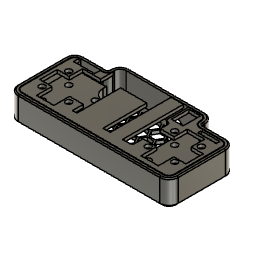
sprig_cover V7 v1 (Autodesk Fusion 360 design; units mm, degrees)
Autodesk Fusion 360 part; units mm, degrees
note: some values were not read from the file. Set by a fixed rule: which sketch regions a step uses.
(part 1 of 2)
sketch "Sketch2" plane through (0, 0, 0) normal (0, 0, 1) x (1, 0, 0)
  line L0 (65.104, -32.4032) -> (-65.104, -32.4032)
  line L1 (70.104, 16.1685) -> (70.104, -27.4032)
  line L2 (70.104, -32.4032) -> (77.8347, -35.9764) construction
  line L3 (12.9089, -32.4032) -> (70.104, -175.9712) construction
  arc A0 (-70.104, -27.4032) -> (-65.104, -32.4032) centre (-65.104, -27.4032) ccw
  line L4 (39.5875, 27.4935) -> (39.6132, 26.0776)
  line L5 (39.4501, 35.0437) -> (39.5, 32.512)
  line L6 (44.6124, 21.1685) -> (65.104, 21.1685)
  arc A1 (39.5875, 27.4935) -> (34.5883, 32.4025) centre (34.5883, 27.4025) ccw
  arc A2 (39.6132, 26.0776) -> (44.6124, 21.1685) centre (44.6124, 26.1685) ccw
  arc A3 (70.104, 16.1685) -> (65.104, 21.1685) centre (65.104, 16.1685) ccw
  arc A4 (65.104, -32.4032) -> (70.104, -27.4032) centre (65.104, -27.4032) ccw
  line L7 (0, 0) -> (0, 41.41)
  arc A5 (-44.6124, 21.1685) -> (-39.6132, 26.0776) centre (-44.6124, 26.1685) ccw
  line L8 (-44.6124, 21.1685) -> (-65.104, 21.1685)
  arc A6 (-65.104, 21.1685) -> (-70.104, 16.1685) centre (-65.104, 16.1685) ccw
  arc A7 (-34.5883, 32.4025) -> (-39.5875, 27.4935) centre (-34.5883, 27.4025) ccw
  line L9 (-39.5875, 27.4935) -> (-39.6132, 26.0776)
  line L10 (-34.5883, 32.4025) -> (34.5883, 32.4025)
  line L11 (-70.104, 16.1685) -> (-70.104, -27.4032)
  arc A8 (40.0874, 27.5026) -> (34.5883, 32.9025) centre (34.5883, 27.4025) ccw
  line L12 (-34.5883, 32.9025) -> (34.5883, 32.9025)
  arc A9 (-34.5883, 32.9025) -> (-40.0874, 27.5026) centre (-34.5883, 27.4025) ccw
  line L13 (-40.0874, 27.5026) -> (-40.1132, 26.0867)
  arc A10 (-44.6124, 21.6685) -> (-40.1132, 26.0867) centre (-44.6124, 26.1685) ccw
  line L14 (-44.6124, 21.6685) -> (-65.104, 21.6685)
  arc A11 (-65.104, 21.6685) -> (-70.604, 16.1685) centre (-65.104, 16.1685) ccw
  line L15 (-70.604, 16.1685) -> (-70.604, -27.4032)
  arc A12 (-70.604, -27.4032) -> (-65.104, -32.9032) centre (-65.104, -27.4032) ccw
  line L16 (65.104, -32.9032) -> (-65.104, -32.9032)
  arc A13 (65.104, -32.9032) -> (70.604, -27.4032) centre (65.104, -27.4032) ccw
  line L17 (70.604, 16.1685) -> (70.604, -27.4032)
  arc A14 (70.604, 16.1685) -> (65.104, 21.6685) centre (65.104, 16.1685) ccw
  line L18 (44.6124, 21.6685) -> (65.104, 21.6685)
  arc A15 (40.1132, 26.0867) -> (44.6124, 21.6685) centre (44.6124, 26.1685) ccw
  line L19 (40.0874, 27.5026) -> (40.1132, 26.0867)
  line L20 (-34.5883, 35.9025) -> (34.5883, 35.9025)
  arc A16 (43.0869, 27.5571) -> (34.5883, 35.9025) centre (34.5883, 27.4025) ccw
  line L21 (43.0869, 27.5571) -> (43.1127, 26.1412)
  arc A17 (43.1127, 26.1412) -> (44.6124, 24.6685) centre (44.6124, 26.1685) ccw
  line L22 (44.6124, 24.6685) -> (65.104, 24.6685)
  arc A18 (73.604, 16.1685) -> (65.104, 24.6685) centre (65.104, 16.1685) ccw
  line L23 (73.604, 16.1685) -> (73.604, -27.4032)
  arc A19 (65.104, -35.9032) -> (73.604, -27.4032) centre (65.104, -27.4032) ccw
  line L24 (65.104, -35.9032) -> (-65.104, -35.9032)
  arc A20 (-73.604, -27.4032) -> (-65.104, -35.9032) centre (-65.104, -27.4032) ccw
  line L25 (-73.604, 16.1685) -> (-73.604, -27.4032)
  arc A21 (-65.104, 24.6685) -> (-73.604, 16.1685) centre (-65.104, 16.1685) ccw
  line L26 (-44.6124, 24.6685) -> (-65.104, 24.6685)
  arc A22 (-44.6124, 24.6685) -> (-43.1127, 26.1412) centre (-44.6124, 26.1685) ccw
  line L27 (-43.0869, 27.5571) -> (-43.1127, 26.1412)
  arc A23 (-34.5883, 35.9025) -> (-43.0869, 27.5571) centre (-34.5883, 27.4025) ccw
  dimension "d1" = 140.208
  dimension "d2" = 65.024
  dimension "d58" = 5
  dimension "d59" = 5
  dimension "d60" = 5
  dimension "d61" = 5
  dimension "d62" = 5
  dimension "d63" = -0.5
  dimension "d64" = 3.5
  constraint horizontal L0
  constraint coincident L2 L7.start
  constraint coincident L3 L7.start
  constraint coincident L7.start origin
  constraint coincident L3.start L0
  constraint tangent L0 A0
  constraint perpendicular L1 L6
  constraint coincident L5.start L4
  constraint tangent L4 A1
  constraint tangent L4 A2
  constraint tangent L6 A2
  constraint coincident L3.end L1
  constraint tangent L6 A3
  constraint tangent L1 A3
  constraint coincident L2.start L0
  constraint coincident L2.start L1
  constraint tangent L0 A4
  constraint tangent L1 A4
  constraint symmetric A1.end L7 A7.start
  constraint symmetric L4.start L7 A7.end
  constraint symmetric A1 L7 A7
  constraint symmetric L4.end L7 A5.end
  constraint symmetric L6.start L7 A5.start
  constraint symmetric A2 L7 A5
  constraint symmetric L6.end L7 L8.end
  constraint symmetric L1.start L7 A6.end
  constraint symmetric A3 L7 A6
  constraint tangent A1 L10
  constraint tangent A0 L11
  measures "d1" distance of L2.end L3.end
  measures "d2" distance of L3.start L2.end
  measures "d58" radius of A0
  measures "d59" radius of A1
  measures "d60" radius of A2
  measures "d61" radius of A3
  measures "d62" radius of A4
sketch "Sketch3" plane through (0, 0, 0) normal (0, 0, 1) x (1, 0, 0)
  line L0 (-70.104, 15.8) -> (-70.104, -27.3)
  arc A0 (-70.104, -27.3) -> (-64.904, -32.5) centre (-64.904, -27.3) ccw
  line L1 (-64.904, -32.5) -> (-30, -32.5)
  arc A1 (-64.904, 21) -> (-70.104, 15.8) centre (-64.904, 15.8) ccw
  line L2 (-64.904, 21) -> (-42, 21)
  line L3 (-30, 9) -> (-30, -32.5)
  circle A2 centre (-30.5373, 18.3875) radius 8
  line L4 (-30.5373, 22.2562) -> (-30.5373, 14.5188)
  line L5 (-42, 21) -> (-42, 19)
  arc A3 (-42, 19) -> (-32, 9) centre (-32, 19) ccw
  line L6 (-32, 9) -> (-30, 9)
  line L7 (0, 0) -> (0, 41.41)
  line L8 (64.904, -32.5) -> (30, -32.5)
  line L9 (30, 9) -> (30, -32.5)
  arc A4 (32, 9) -> (42, 19) centre (32, 19) ccw
  line L10 (64.904, 21) -> (42, 21)
  line L11 (42, 21) -> (42, 19)
  line L12 (70.104, 15.8) -> (70.104, -27.3)
  arc A5 (70.104, 15.8) -> (64.904, 21) centre (64.904, 15.8) ccw
  arc A6 (64.904, -32.5) -> (70.104, -27.3) centre (64.904, -27.3) ccw
  line L13 (30, 9) -> (32, 9)
  line L14 (-64.904, -27.5) -> (-35, -27.5)
  line L15 (-35, 4.3031) -> (-35, -27.5)
  arc A7 (-46.6969, 16) -> (-35, 4.3031) centre (-32, 19) ccw
  line L16 (-64.904, 16) -> (-46.6969, 16)
  arc A8 (-64.904, 16) -> (-65.104, 15.8) centre (-64.904, 15.8) ccw
  line L17 (-65.104, 15.8) -> (-65.104, -27.3)
  arc A9 (-65.104, -27.3) -> (-64.904, -27.5) centre (-64.904, -27.3) ccw
  line L18 (64.904, -27.5) -> (35, -27.5)
  line L19 (35, 4.3031) -> (35, -27.5)
  arc A10 (35, 4.3031) -> (46.6969, 16) centre (32, 19) ccw
  line L20 (64.904, 16) -> (46.6969, 16)
  arc A11 (65.104, 15.8) -> (64.904, 16) centre (64.904, 15.8) ccw
  line L21 (65.104, 15.8) -> (65.104, -27.3)
  arc A12 (64.904, -27.5) -> (65.104, -27.3) centre (64.904, -27.3) ccw
  dimension "d3" = 70.104
  dimension "d4" = 32.5
  dimension "d5" = 5.2
  dimension "d6" = 21
  dimension "d7" = 5.2
  dimension "d8" = 16
  dimension "d9" = 42
  dimension "d10" = 9
  dimension "d11" = 10
  dimension "d12" = 30
  dimension "d97" = 5
  dimension "d98" = -5
  constraint vertical L0
  constraint tangent L0 A0
  constraint horizontal L1
  constraint tangent A0 L1
  constraint tangent L0 A1
  constraint horizontal L2
  constraint tangent A1 L2
  constraint perpendicular L2 L3
  constraint coincident L1.end L3.end
  constraint vertical L4
  constraint midpoint A2.centre L4
  constraint perpendicular L2 L5
  constraint tangent L5 A3
  constraint perpendicular L5 L6
  constraint tangent A3 L6
  constraint symmetric L0.start L7 L12.start
  constraint symmetric L0.end L7 L12.end
  constraint symmetric A0.end L7 L8.start
  constraint symmetric A0 L7 A6
  constraint symmetric L1.end L7 L8.end
  constraint symmetric A1.start L7 L10.start
  constraint symmetric A1 L7 A5
  constraint symmetric L2.end L7 L10.end
  constraint symmetric L5.end L7 A4.end
  constraint symmetric A3.end L7 A4.start
  constraint symmetric A3 L7 A4
  constraint symmetric L3.start L7 L9.start
  measures "d3" distance of L7.start L0
  measures "d4" distance of L7.start L1
  measures "d5" radius of A0
  measures "d6" distance of L7.start L2
  measures "d7" radius of A1
  measures "d8" diameter of A2
  measures "d9" distance of L7.start L5
  measures "d10" distance of L7.start L6
  measures "d11" radius of A3
  measures "d12" distance of L7.start L3
extrude "Extrude1" add sketch "Sketch3" against normal blind 4 contours L0 A0 L1 A1 L2 L3 L5 A3 L6 | L14 L15 A7 L16 A8 L17 A9 makes body 1
fillet "Fillet3" radius 1 3 edges at (-30, -32.5, -2) (-30, 9, -2) (-42, 21, -2) on bodies 1
pattern_linear "R-Pattern1" count 2 spacing 4 along (0, 0, -1) of bodies 1 makes body 2
sketch "Sketch4" plane through (0, 0, 0) normal (0, 0, 1) x (-1, 0, 0)
  arc A0 (64.904, -21) -> (70.104, -15.8) centre (64.904, -15.8) ccw
  line L0 (70.104, -15.8) -> (70.104, 27.3)
  arc A1 (70.104, 27.3) -> (64.904, 32.5) centre (64.904, 27.3) ccw
  line L1 (64.904, 32.5) -> (31, 32.5)
  line L2 (30, 31.5) -> (30, -8)
  line L3 (31, -9) -> (32, -9)
  arc A2 (42, -19) -> (32, -9) centre (32, -19) ccw
  line L4 (42, -19) -> (42, -20)
  line L5 (43, -21) -> (64.904, -21)
  line L6 (65.35, -2.7) -> (48.35, -2.7)
  line L7 (65.35, 14.3) -> (65.35, -2.7)
  arc A3 (42, -20) -> (43, -21) centre (43, -20) ccw
  arc A4 (31, 32.5) -> (30, 31.5) centre (31, 31.5) ccw
  arc A5 (30, -8) -> (31, -9) centre (31, -8) ccw
  point P0 (48.35, 5.8)
  dimension "d21" = 5.8
  dimension "d23" = 48.35
  dimension "d24" = 17
  constraint horizontal L6
  constraint vertical L7
  measures "d21" vertical distance of origin P0
  measures "d23" horizontal distance of origin P0
  measures "d24" distance of L6.start L7.start
sketch "Sketch5" plane through (0, 0, 0) normal (0, 0, 1) x (-1, 0, 0)
  arc A0 (42, -20) -> (43, -21) centre (43, -20) ccw
  line L0 (43, -21) -> (64.904, -21)
  arc A1 (64.904, -21) -> (70.104, -15.8) centre (64.904, -15.8) ccw
  line L1 (70.104, -15.8) -> (70.104, 27.3)
  arc A2 (70.104, 27.3) -> (64.904, 32.5) centre (64.904, 27.3) ccw
  line L2 (64.904, 32.5) -> (31, 32.5)
  arc A3 (31, 32.5) -> (30, 31.5) centre (31, 31.5) ccw
  line L3 (30, 31.5) -> (30, -8)
  arc A4 (30, -8) -> (31, -9) centre (31, -8) ccw
  line L4 (31, -9) -> (32, -9)
  arc A5 (42, -19) -> (32, -9) centre (32, -19) ccw
  line L5 (42, -19) -> (42, -20)
  line L6 (62.35, -2.7) -> (62.35, -15.2)
  line L7 (62.35, -15.2) -> (51.35, -15.2)
  line L8 (51.35, -15.2) -> (51.35, -2.7)
  point P0 (56.85, -2.7)
  point P1 (56.85, -15.2)
  dimension "d37" = 12.5
  dimension "d38" = 11
  constraint perpendicular L6 L7
  constraint midpoint L7 P1
  constraint vertical P0 P1
  measures "d37" distance of L7.end L8.end
  measures "d38" distance of L6.end L7.end
sketch "Sketch6" plane through (0, 0, 0) normal (0, 0, 1) x (-1, 0, 0)
  arc A0 (42, -20) -> (43, -21) centre (43, -20) ccw
  line L0 (43, -21) -> (64.904, -21)
  arc A1 (64.904, -21) -> (70.104, -15.8) centre (64.904, -15.8) ccw
  line L1 (70.104, -15.8) -> (70.104, 27.3)
  arc A2 (70.104, 27.3) -> (64.904, 32.5) centre (64.904, 27.3) ccw
  line L2 (64.904, 32.5) -> (31, 32.5)
  arc A3 (31, 32.5) -> (30, 31.5) centre (31, 31.5) ccw
  line L3 (30, 31.5) -> (30, -8)
  arc A4 (30, -8) -> (31, -9) centre (31, -8) ccw
  line L4 (31, -9) -> (32, -9)
  arc A5 (42, -19) -> (32, -9) centre (32, -19) ccw
  line L5 (42, -19) -> (42, -20)
  circle A6 centre (60.5272, -6.0993) radius 1.1
  circle A7 centre (36.0826, -6.0993) radius 1.1
  line L6 (60.5272, -6.0993) -> (36.0826, -6.0993) construction
  line L7 (36.0826, -6.0993) -> (36.0826, 18.3161) construction
  line L8 (36.0826, 18.3161) -> (60.5272, 18.3161) construction
  line L9 (60.5272, 18.3161) -> (60.5272, -6.0993) construction
  circle A8 centre (60.5272, 18.3161) radius 1.1
  circle A9 centre (36.0826, 18.3161) radius 1.1
  dimension "d45" = 2.2
  dimension "d46" = 2.2
  dimension "d47" = 2.2
  dimension "d48" = 2.2
  constraint horizontal L6
  constraint vertical L7
  constraint horizontal L8
  constraint vertical L9
  constraint coincident A6.centre L6.start
  constraint coincident A7.centre L6.end
  constraint coincident L8.end L9.start
  constraint coincident L7.end L8.start
  measures "d45" diameter of A6
  measures "d46" diameter of A7
  measures "d47" diameter of A8
  measures "d48" diameter of A9
sketch "Sketch10" plane through (0, 0, 0) normal (0, 0, 1) x (-1, 0, 0)
  arc A0 (42, -20) -> (43, -21) centre (43, -20) ccw
  line L0 (43, -21) -> (64.904, -21)
  arc A1 (64.904, -21) -> (70.104, -15.8) centre (64.904, -15.8) ccw
  line L1 (70.104, -15.8) -> (70.104, 27.3)
  arc A2 (70.104, 27.3) -> (64.904, 32.5) centre (64.904, 27.3) ccw
  line L2 (64.904, 32.5) -> (31, 32.5)
  arc A3 (31, 32.5) -> (30, 31.5) centre (31, 31.5) ccw
  line L3 (30, 31.5) -> (30, -8)
  arc A4 (30, -8) -> (31, -9) centre (31, -8) ccw
  line L4 (31, -9) -> (32, -9)
  arc A5 (42, -19) -> (32, -9) centre (32, -19) ccw
  line L5 (42, -19) -> (42, -20)
sketch "Sketch11" plane through (0, 0, -4) normal (0, 0, 1) x (-1, 0, 0)
  arc A0 (42, -20) -> (43, -21) centre (43, -20) ccw
  line L0 (43, -21) -> (64.904, -21)
  arc A1 (64.904, -21) -> (70.104, -15.8) centre (64.904, -15.8) ccw
  line L1 (70.104, -15.8) -> (70.104, 27.3)
  arc A2 (70.104, 27.3) -> (64.904, 32.5) centre (64.904, 27.3) ccw
  line L2 (64.904, 32.5) -> (31, 32.5)
  arc A3 (31, 32.5) -> (30, 31.5) centre (31, 31.5) ccw
  line L3 (30, 31.5) -> (30, -8)
  arc A4 (30, -8) -> (31, -9) centre (31, -8) ccw
  line L4 (31, -9) -> (32, -9)
  arc A5 (42, -19) -> (32, -9) centre (32, -19) ccw
  line L5 (42, -19) -> (42, -20)
extrude "Extrude7" add sketch "Sketch2" along normal blind 7 separate body contours L20 A16 L21 A17 L22 A18 L23 A19 L24 A20 L25 A21 L26 A22 L27 A23 makes body 3
extrude "Extrude8" add 1 faces at (-21.7013, -33.9032, 0) along direction (0, 0, -1) blind 18 separate body on bodies 3 makes body 4
extrude "Extrude9" add sketch "Sketch3" against normal blind 7.75 separate body contours A2 makes body 5
sketch "Sketch12" plane through (0, 0, -18) normal (0, 0, -1) x (1, 0, 0)
  arc A0 (-40.0874, -27.5026) -> (-34.5883, -32.9025) centre (-34.5883, -27.4025) ccw
  line L0 (-40.0874, -27.5026) -> (-40.1132, -26.0867)
  arc A1 (-40.1132, -26.0867) -> (-44.6124, -21.6685) centre (-44.6124, -26.1685) ccw
  line L1 (-44.6124, -21.6685) -> (-65.104, -21.6685)
  arc A2 (-70.604, -16.1685) -> (-65.104, -21.6685) centre (-65.104, -16.1685) ccw
  line L2 (-70.604, -16.1685) -> (-70.604, 27.4032)
  arc A3 (-65.104, 32.9032) -> (-70.604, 27.4032) centre (-65.104, 27.4032) ccw
  line L3 (-65.104, 32.9032) -> (65.104, 32.9032)
  arc A4 (70.604, 27.4032) -> (65.104, 32.9032) centre (65.104, 27.4032) ccw
  line L4 (70.604, 27.4032) -> (70.604, -16.1685)
  arc A5 (65.104, -21.6685) -> (70.604, -16.1685) centre (65.104, -16.1685) ccw
  line L5 (65.104, -21.6685) -> (44.6124, -21.6685)
  arc A6 (44.6124, -21.6685) -> (40.1132, -26.0867) centre (44.6124, -26.1685) ccw
  line L6 (40.1132, -26.0867) -> (40.0874, -27.5026)
  arc A7 (34.5883, -32.9025) -> (40.0874, -27.5026) centre (34.5883, -27.4025) ccw
  line L7 (34.5883, -32.9025) -> (-34.5883, -32.9025)
  arc A8 (34.5883, -35.9025) -> (43.0869, -27.5571) centre (34.5883, -27.4025) ccw
  line L8 (43.0869, -27.5571) -> (43.1127, -26.1412)
  arc A9 (44.6124, -24.6685) -> (43.1127, -26.1412) centre (44.6124, -26.1685) ccw
  line L9 (44.6124, -24.6685) -> (65.104, -24.6685)
  arc A10 (65.104, -24.6685) -> (73.604, -16.1685) centre (65.104, -16.1685) ccw
  line L10 (73.604, -16.1685) -> (73.604, 27.4032)
  arc A11 (73.604, 27.4032) -> (65.104, 35.9032) centre (65.104, 27.4032) ccw
  line L11 (65.104, 35.9032) -> (-65.104, 35.9032)
  arc A12 (-65.104, 35.9032) -> (-73.604, 27.4032) centre (-65.104, 27.4032) ccw
  line L12 (-73.604, 27.4032) -> (-73.604, -16.1685)
  arc A13 (-73.604, -16.1685) -> (-65.104, -24.6685) centre (-65.104, -16.1685) ccw
  line L13 (-65.104, -24.6685) -> (-44.6124, -24.6685)
  arc A14 (-43.1127, -26.1412) -> (-44.6124, -24.6685) centre (-44.6124, -26.1685) ccw
  line L14 (-43.1127, -26.1412) -> (-43.0869, -27.5571)
  arc A15 (-43.0869, -27.5571) -> (-34.5883, -35.9025) centre (-34.5883, -27.4025) ccw
  line L15 (-34.5883, -35.9025) -> (34.5883, -35.9025)
  line L16 (65.104, 35.9032) -> (-65.104, 35.9032)
  arc A16 (-65.104, 35.9032) -> (-73.604, 27.4032) centre (-65.104, 27.4032) ccw
  line L17 (-73.604, -16.1685) -> (-73.604, 27.4032)
  arc A17 (-73.604, -16.1685) -> (-65.104, -24.6685) centre (-65.104, -16.1685) ccw
  line L18 (-44.6124, -24.6685) -> (-65.104, -24.6685)
  line L19 (-34.5883, -35.9025) -> (34.5883, -35.9025)
  arc A18 (-43.0869, -27.5571) -> (-34.5883, -35.9025) centre (-34.5883, -27.4025) ccw
  arc A19 (-43.1127, -26.1412) -> (-44.6124, -24.6685) centre (-44.6124, -26.1685) ccw
  line L20 (-43.0869, -27.5571) -> (-43.1127, -26.1412)
  arc A20 (34.5883, -35.9025) -> (43.0869, -27.5571) centre (34.5883, -27.4025) ccw
  line L21 (44.6124, -24.6685) -> (65.104, -24.6685)
  line L22 (43.0869, -27.5571) -> (43.1127, -26.1412)
  arc A21 (44.6124, -24.6685) -> (43.1127, -26.1412) centre (44.6124, -26.1685) ccw
  arc A22 (65.104, -24.6685) -> (73.604, -16.1685) centre (65.104, -16.1685) ccw
  line L23 (73.604, -16.1685) -> (73.604, 27.4032)
  arc A23 (73.604, 27.4032) -> (65.104, 35.9032) centre (65.104, 27.4032) ccw
extrude "Extrude10" add sketch "Sketch12" along normal blind 3 separate body contours A0 L0 A1 L1 A2 L2 A3 L3 A4 L4 A5 L5 A6 L6 A7 L7 | A8 L8 A9 L9 A10 L10 A11 L11 A12 L12 A13 L13 A14 L14 A15 L15 L16 A16 L17 A17 L18 L19 A18 A19 L20 A20 L21 L22 A21 A22 L23 A23 makes body 6
sketch "Sketch13" plane through (0, 0, -8) normal (0, 0, -1) x (1, 0, 0)
  arc A0 (-43, -21) -> (-42, -20) centre (-43, -20) ccw
  line L0 (-42, -20) -> (-42, -19)
  arc A1 (-32, -9) -> (-42, -19) centre (-32, -19) ccw
  line L1 (-32, -9) -> (-31, -9)
  arc A2 (-31, -9) -> (-30, -8) centre (-31, -8) ccw
  line L2 (-30, -8) -> (-30, 31.5)
  arc A3 (-30, 31.5) -> (-31, 32.5) centre (-31, 31.5) ccw
  line L3 (-31, 32.5) -> (-64.904, 32.5)
  arc A4 (-64.904, 32.5) -> (-70.104, 27.3) centre (-64.904, 27.3) ccw
  line L4 (-70.104, 27.3) -> (-70.104, -15.8)
  arc A5 (-70.104, -15.8) -> (-64.904, -21) centre (-64.904, -15.8) ccw
  line L5 (-64.904, -21) -> (-43, -21)
  line L6 (0, -40) -> (0, 40)
  line L7 (42, -20) -> (42, -19)
  arc A6 (30, -8) -> (31, -9) centre (31, -8) ccw
  line L8 (70.104, 27.3) -> (70.104, -15.8)
  arc A7 (42, -20) -> (43, -21) centre (43, -20) ccw
  line L9 (32, -9) -> (31, -9)
  line L10 (30, -8) -> (30, 31.5)
  line L11 (31, 32.5) -> (64.904, 32.5)
  arc A8 (70.104, 27.3) -> (64.904, 32.5) centre (64.904, 27.3) ccw
  arc A9 (31, 32.5) -> (30, 31.5) centre (31, 31.5) ccw
  arc A10 (64.904, -21) -> (70.104, -15.8) centre (64.904, -15.8) ccw
  line L12 (64.904, -21) -> (43, -21)
  arc A11 (42, -19) -> (32, -9) centre (32, -19) ccw
  line L13 (30, -8) -> (30, -32.9025)
  line L14 (-34.5883, -32.4025) -> (34.5883, -32.4025)
  arc A12 (34.5883, -32.4025) -> (39.5875, -27.4935) centre (34.5883, -27.4025) ccw
  arc A13 (44.6124, -21.1685) -> (39.6132, -26.0776) centre (44.6124, -26.1685) ccw
  line L15 (39.5875, -27.4935) -> (39.6132, -26.0776)
  line L16 (42, -19.5) -> (42, -21.9053)
  line L17 (45.6567, -21) -> (44.6124, -21.1685)
  arc A14 (-40.0874, -27.5026) -> (-34.5883, -32.9025) centre (-34.5883, -27.4025) ccw
  line L18 (-34.5883, -32.9025) -> (34.5883, -32.9025)
  arc A15 (34.5883, -32.9025) -> (40.0874, -27.5026) centre (34.5883, -27.4025) ccw
  line L19 (40.0874, -27.5026) -> (40.1132, -26.0867)
  arc A16 (44.6124, -21.6685) -> (40.1132, -26.0867) centre (44.6124, -26.1685) ccw
  line L20 (44.6124, -21.6685) -> (65.104, -21.6685)
  arc A17 (65.104, -21.6685) -> (70.604, -16.1685) centre (65.104, -16.1685) ccw
  line L21 (70.604, -16.1685) -> (70.604, 27.4032)
  arc A18 (70.604, 27.4032) -> (65.104, 32.9032) centre (65.104, 27.4032) ccw
  line L22 (65.104, 32.9032) -> (-65.104, 32.9032)
  arc A19 (-65.104, 32.9032) -> (-70.604, 27.4032) centre (-65.104, 27.4032) ccw
  line L23 (-70.604, 27.4032) -> (-70.604, -16.1685)
  arc A20 (-70.604, -16.1685) -> (-65.104, -21.6685) centre (-65.104, -16.1685) ccw
  line L24 (-65.104, -21.6685) -> (-44.6124, -21.6685)
  arc A21 (-40.1132, -26.0867) -> (-44.6124, -21.6685) centre (-44.6124, -26.1685) ccw
  line L25 (-40.1132, -26.0867) -> (-40.0874, -27.5026)
  arc A22 (34.5883, -35.9025) -> (43.0869, -27.5571) centre (34.5883, -27.4025) ccw
  line L26 (34.5883, -35.9025) -> (-34.5883, -35.9025)
  arc A23 (-43.0869, -27.5571) -> (-34.5883, -35.9025) centre (-34.5883, -27.4025) ccw
  line L27 (-43.0869, -27.5571) -> (-43.1127, -26.1412)
  arc A24 (-43.1127, -26.1412) -> (-44.6124, -24.6685) centre (-44.6124, -26.1685) ccw
  line L28 (-44.6124, -24.6685) -> (-65.104, -24.6685)
  arc A25 (-73.604, -16.1685) -> (-65.104, -24.6685) centre (-65.104, -16.1685) ccw
  line L29 (-73.604, -16.1685) -> (-73.604, 27.4032)
  arc A26 (-65.104, 35.9032) -> (-73.604, 27.4032) centre (-65.104, 27.4032) ccw
  line L30 (-65.104, 35.9032) -> (65.104, 35.9032)
  arc A27 (73.604, 27.4032) -> (65.104, 35.9032) centre (65.104, 27.4032) ccw
  line L31 (73.604, 27.4032) -> (73.604, -16.1685)
  arc A28 (65.104, -24.6685) -> (73.604, -16.1685) centre (65.104, -16.1685) ccw
  line L32 (65.104, -24.6685) -> (44.6124, -24.6685)
  arc A29 (44.6124, -24.6685) -> (43.1127, -26.1412) centre (44.6124, -26.1685) ccw
  line L33 (43.1127, -26.1412) -> (43.0869, -27.5571)
  line L34 (-42, -19) -> (-42, -22.5045)
  line L35 (-30, 31.5) -> (-30, 32.9032)
  line L36 (30, 31.5) -> (30, 32.9032)
  constraint vertical L6
  constraint symmetric A0.start L6 A7.end
  constraint symmetric A0.end L6 L7.start
  constraint symmetric A0 L6 A7
  constraint symmetric L0.end L6 L7.end
  constraint symmetric A1.start L6 L9.start
  constraint symmetric A1 L6 A11
  constraint symmetric L1.end L6 A6.end
  constraint symmetric A2.end L6 A6.start
  constraint symmetric A2 L6 A6
  constraint symmetric L2.end L6 L10.end
  constraint symmetric A3.end L6 L11.start
  constraint symmetric A3 L6 A9
  constraint symmetric L3.end L6 L11.end
  constraint symmetric A4.end L6 L8.start
  constraint symmetric A4 L6 A8
  constraint symmetric L4.end L6 L8.end
  constraint symmetric A5.end L6 A10.start
  constraint symmetric A5 L6 A10
  constraint tangent A6 L13
  constraint midpoint L7 L16.start
  constraint coincident A13 L16.end
  constraint parallel L7 L16
  constraint coincident L12 L17.start
  constraint coincident A13.start L17.end
  constraint coincident L0.end A1.end
  constraint coincident A21 L34.end
  constraint tangent A1 L34
  constraint coincident L2.end A3.start
  constraint coincident L22 L35.end
  constraint tangent A3 L35
  constraint coincident L22 L36.end
  constraint tangent A9 L36
  constraint coincident L13.end L18
extrude "Extrude11" add sketch "Sketch13" along normal up to surface (10 mm away) separate body contours A0 L0 A1 L1 A2 L2 A3 L3 A4 L4 A5 L5 L34 | A0 A3 L3 A4 L4 A5 L5 L22 A19 L23 A20 L24 A21 L34 L35 | L8 L11 A8 A9 A10 L12 L13 L14 A12 A13 L15 L17 L18 A15 L19 A16 L20 A17 L21 A18 L22 L36 | L7 A6 L9 A11 L13 L14 A12 A13 L15 L16 | L7 A6 L8 A7 L9 L10 L11 A8 A9 A10 L12 A11 L16 | A7 L12 A13 L16 L17 makes body 7 at (-43.7527, -18.6342, -8) makes body 8 at (48.4055, -12.8793, -18)
sketch "Sketch15" plane through (0, 0, -8) normal (0, 0, 1) x (-1, 0, 0)
  arc A0 (-54.9753, -18.5428) -> (-41.9871, -20.3021) centre (-48.0353, -16.1308) ccw
  line L0 (-41.9871, -20.3021) -> (-41.9873, -19.0036)
  arc A1 (-32.0015, -9.0019) -> (-41.9873, -19.0036) centre (-31.9919, -18.9973) ccw
  line L1 (-32.0015, -9.0019) -> (-30.9998, -9.0018)
  arc A2 (-30.9998, -9.0018) -> (-29.9996, -8.0003) centre (-31.0003, -8.001) ccw
  line L2 (-29.9996, -8.0003) -> (-30.0003, 31.5)
  arc A3 (-30.0003, 31.5) -> (-31, 32.4989) centre (-30.9998, 31.4994) ccw
  line L3 (-31, 32.4989) -> (-64.904, 32.4966)
  arc A4 (-64.904, 32.4966) -> (-70.0751, 27.2999) centre (-64.8897, 27.3112) ccw
  line L4 (-70.0751, 27.2999) -> (-70.4263, -15.7823)
  arc A5 (-70.4263, -15.7823) -> (-55.331, -20.7119) centre (-62.9093, -18.3409) ccw
  line L5 (-55.331, -20.7119) -> (-54.9753, -18.5428)
  circle A6 centre (60.5404, -6.0319) radius 2.75
  circle A7 centre (36.0404, -6.0319) radius 2.75
  circle A8 centre (60.5404, 18.4681) radius 2.75
  circle A9 centre (36.0404, 18.4681) radius 2.75
  line L6 (0, 0) -> (0, -24.1722)
  circle A10 centre (-60.5404, 17.4681) radius 2.75
  circle A11 centre (-36.0404, 17.4681) radius 2.75
  circle A12 centre (-36.0404, -7.0319) radius 2.75
  circle A13 centre (-60.5404, -7.0319) radius 2.75
  line L7 (-30, -32.9025) -> (-30, 32.9032)
  line L8 (-30, -32.9025) -> (-30.1, -32.4)
  arc A14 (-39.5875, -27.4935) -> (-34.5883, -32.4025) centre (-34.5883, -27.4025) ccw
  line L9 (34.5883, -32.4025) -> (-34.5883, -32.4025)
  arc A15 (-39.6132, -26.0776) -> (-44.6124, -21.1685) centre (-44.6124, -26.1685) ccw
  line L10 (-39.5875, -27.4935) -> (-39.6132, -26.0776)
  line L11 (-45.6567, -21) -> (-43, -21.4357)
  line L12 (-30, 32.9032) -> (-65.104, 32.9032)
  arc A16 (-65.104, 32.9032) -> (-70.604, 27.4032) centre (-65.104, 27.4032) ccw
  line L13 (-70.604, 27.4032) -> (-70.604, -16.1685)
  arc A17 (-70.604, -16.1685) -> (-65.104, -21.6685) centre (-65.104, -16.1685) ccw
  line L14 (-65.104, -21.6685) -> (-44.6124, -21.6685)
  arc A18 (-40.1132, -26.0867) -> (-44.6124, -21.6685) centre (-44.6124, -26.1685) ccw
  line L15 (-40.1132, -26.0867) -> (-40.0874, -27.5026)
  arc A19 (-40.0874, -27.5026) -> (-34.5883, -32.9025) centre (-34.5883, -27.4025) ccw
  line L16 (-34.5883, -32.9025) -> (-30, -32.9025)
  dimension "d76" = 5.5
  dimension "d79" = -24.5
  dimension "d80" = 24.5
  constraint coincident L6.start origin
  constraint vertical L6
  constraint coincident L7.start L8.start
  constraint coincident A15 L11.end
  constraint perpendicular L5 L11
  measures "d76" diameter of A6
extrude "Extrude12" cut sketch "Sketch15" against normal blind 5 contours A1 A12 | A1 A12 | A6 | A7 | A8 | A9 | A10 | A11 | A13 bodies 7 8
sketch "Sketch16" plane through (0, 0, -21) normal (0, 0, -1) x (1, 0, 0)
  line L0 (44.6124, -24.6685) -> (65.104, -24.6685)
  arc A0 (65.104, -24.6685) -> (73.604, -16.1685) centre (65.104, -16.1685) ccw
  line L1 (73.604, -16.1685) -> (73.604, 27.4032)
  arc A1 (73.604, 27.4032) -> (65.104, 35.9032) centre (65.104, 27.4032) ccw
  line L2 (65.104, 35.9032) -> (-65.104, 35.9032)
  arc A2 (-65.104, 35.9032) -> (-73.604, 27.4032) centre (-65.104, 27.4032) ccw
  line L3 (-73.604, 27.4032) -> (-73.604, -16.1685)
  arc A3 (-73.604, -16.1685) -> (-65.104, -24.6685) centre (-65.104, -16.1685) ccw
  line L4 (-65.104, -24.6685) -> (-44.6124, -24.6685)
  arc A4 (-43.1127, -26.1412) -> (-44.6124, -24.6685) centre (-44.6124, -26.1685) ccw
  line L5 (-43.1127, -26.1412) -> (-43.0869, -27.5571)
  arc A5 (-43.0869, -27.5571) -> (-34.5883, -35.9025) centre (-34.5883, -27.4025) ccw
  line L6 (-34.5883, -35.9025) -> (34.5883, -35.9025)
  arc A6 (34.5883, -35.9025) -> (43.0869, -27.5571) centre (34.5883, -27.4025) ccw
  line L7 (43.0869, -27.5571) -> (43.1127, -26.1412)
  arc A7 (44.6124, -24.6685) -> (43.1127, -26.1412) centre (44.6124, -26.1685) ccw
  line L8 (-30, -8) -> (-30, 31.5)
  arc A8 (-32, -9) -> (-42, -19) centre (-32, -19) ccw
  line L9 (-43, -21) -> (-64.904, -21)
  arc A9 (-70.104, -15.8) -> (-64.904, -21) centre (-64.904, -15.8) ccw
  arc A10 (42, -19) -> (32, -9) centre (32, -19) ccw
  line L10 (30, -8) -> (30, 31.5)
  line L11 (64.904, -21) -> (43, -21)
  line L12 (70.104, 27.3) -> (70.104, -15.8)
  line L13 (31, 32.5) -> (64.904, 32.5)
  line L14 (-2.8868, 5) -> (-5.7735, 0)
  line L15 (-5.7735, 0) -> (-2.8868, -5)
  line L16 (-2.8868, -5) -> (2.8868, -5)
  line L17 (2.8868, -5) -> (5.7735, 0)
  line L18 (5.7735, 0) -> (2.8868, 5)
  line L19 (2.8868, 5) -> (-2.8868, 5)
  line L20 (0, 0) -> (0, 5)
  line L21 (0, 0) -> (2.8868, 5)
  line L22 (32.8868, -35.0385) -> (27.1132, -35.0385)
  line L23 (37.1132, -27.718) -> (42.8868, -27.718)
  line L24 (34.2265, -22.718) -> (37.1132, -27.718)
  line L25 (37.1132, -17.718) -> (34.2265, -22.718)
  line L26 (42.8868, -17.718) -> (37.1132, -17.718)
  line L27 (42.8868, -27.718) -> (45.7735, -22.718)
  line L28 (45.7735, -22.718) -> (42.8868, -17.718)
  line L29 (27.1132, -33.5385) -> (32.8868, -33.5385)
  line L30 (24.2265, -28.5385) -> (27.1132, -33.5385)
  line L31 (27.1132, -23.5385) -> (24.2265, -28.5385)
  line L32 (32.8868, -23.5385) -> (27.1132, -23.5385)
  line L33 (32.8868, -33.5385) -> (35.7735, -28.5385)
  line L34 (35.7735, -28.5385) -> (32.8868, -23.5385)
  line L35 (37.1132, -16.218) -> (42.8868, -16.218)
  line L36 (34.2265, -11.218) -> (37.1132, -16.218)
  line L37 (37.1132, -6.218) -> (34.2265, -11.218)
  line L38 (42.8868, -6.218) -> (37.1132, -6.218)
  line L39 (42.8868, -16.218) -> (45.7735, -11.218)
  line L40 (45.7735, -11.218) -> (42.8868, -6.218)
  line L41 (17.1132, -29.359) -> (14.2265, -34.359)
  line L42 (22.8868, -29.359) -> (17.1132, -29.359)
  line L43 (25.7735, -34.359) -> (22.8868, -29.359)
  line L44 (27.1132, -22.0385) -> (32.8868, -22.0385)
  line L45 (24.2265, -17.0385) -> (27.1132, -22.0385)
  line L46 (27.1132, -12.0385) -> (24.2265, -17.0385)
  line L47 (32.8868, -12.0385) -> (27.1132, -12.0385)
  line L48 (32.8868, -22.0385) -> (35.7735, -17.0385)
  line L49 (35.7735, -17.0385) -> (32.8868, -12.0385)
  line L50 (37.1132, -4.718) -> (42.8868, -4.718)
  line L51 (34.2265, 0.282) -> (37.1132, -4.718)
  line L52 (37.1132, 5.282) -> (34.2265, 0.282)
  line L53 (42.8868, 5.282) -> (37.1132, 5.282)
  line L54 (42.8868, -4.718) -> (45.7735, 0.282)
  line L55 (45.7735, 0.282) -> (42.8868, 5.282)
  line L56 (12.8868, -35.1795) -> (7.1132, -35.1795)
  line L57 (17.1132, -27.859) -> (22.8868, -27.859)
  line L58 (14.2265, -22.859) -> (17.1132, -27.859)
  line L59 (17.1132, -17.859) -> (14.2265, -22.859)
  line L60 (22.8868, -17.859) -> (17.1132, -17.859)
  line L61 (22.8868, -27.859) -> (25.7735, -22.859)
  line L62 (25.7735, -22.859) -> (22.8868, -17.859)
  line L63 (27.1132, -10.5385) -> (32.8868, -10.5385)
  line L64 (24.2265, -5.5385) -> (27.1132, -10.5385)
  line L65 (27.1132, -0.5385) -> (24.2265, -5.5385)
  line L66 (32.8868, -0.5385) -> (27.1132, -0.5385)
  line L67 (32.8868, -10.5385) -> (35.7735, -5.5385)
  line L68 (35.7735, -5.5385) -> (32.8868, -0.5385)
  line L69 (37.1132, 6.782) -> (42.8868, 6.782)
  line L70 (34.2265, 11.782) -> (37.1132, 6.782)
  line L71 (37.1132, 16.782) -> (34.2265, 11.782)
  line L72 (42.8868, 16.782) -> (37.1132, 16.782)
  line L73 (42.8868, 6.782) -> (45.7735, 11.782)
  line L74 (45.7735, 11.782) -> (42.8868, 16.782)
  line L75 (7.1132, -33.6795) -> (12.8868, -33.6795)
  line L76 (4.2265, -28.6795) -> (7.1132, -33.6795)
  line L77 (7.1132, -23.6795) -> (4.2265, -28.6795)
  line L78 (12.8868, -23.6795) -> (7.1132, -23.6795)
  line L79 (12.8868, -33.6795) -> (15.7735, -28.6795)
  line L80 (15.7735, -28.6795) -> (12.8868, -23.6795)
  line L81 (17.1132, -16.359) -> (22.8868, -16.359)
  line L82 (14.2265, -11.359) -> (17.1132, -16.359)
  line L83 (17.1132, -6.359) -> (14.2265, -11.359)
  line L84 (22.8868, -6.359) -> (17.1132, -6.359)
  line L85 (22.8868, -16.359) -> (25.7735, -11.359)
  line L86 (25.7735, -11.359) -> (22.8868, -6.359)
  line L87 (27.1132, 0.9615) -> (32.8868, 0.9615)
  line L88 (24.2265, 5.9615) -> (27.1132, 0.9615)
  line L89 (27.1132, 10.9615) -> (24.2265, 5.9615)
  line L90 (32.8868, 10.9615) -> (27.1132, 10.9615)
  line L91 (32.8868, 0.9615) -> (35.7735, 5.9615)
  line L92 (35.7735, 5.9615) -> (32.8868, 10.9615)
  line L93 (37.1132, 18.282) -> (42.8868, 18.282)
  line L94 (34.2265, 23.282) -> (37.1132, 18.282)
  line L95 (37.1132, 28.282) -> (34.2265, 23.282)
  line L96 (42.8868, 28.282) -> (37.1132, 28.282)
  line L97 (42.8868, 18.282) -> (45.7735, 23.282)
  line L98 (45.7735, 23.282) -> (42.8868, 28.282)
  line L99 (-2.8868, -29.5) -> (-5.7735, -34.5)
  line L100 (2.8868, -29.5) -> (-2.8868, -29.5)
  line L101 (5.7735, -34.5) -> (2.8868, -29.5)
  line L102 (7.1132, -22.1795) -> (12.8868, -22.1795)
  line L103 (4.2265, -17.1795) -> (7.1132, -22.1795)
  line L104 (7.1132, -12.1795) -> (4.2265, -17.1795)
  line L105 (12.8868, -12.1795) -> (7.1132, -12.1795)
  line L106 (12.8868, -22.1795) -> (15.7735, -17.1795)
  line L107 (15.7735, -17.1795) -> (12.8868, -12.1795)
  line L108 (17.1132, -4.859) -> (22.8868, -4.859)
  line L109 (14.2265, 0.141) -> (17.1132, -4.859)
  line L110 (17.1132, 5.141) -> (14.2265, 0.141)
  line L111 (22.8868, 5.141) -> (17.1132, 5.141)
  line L112 (22.8868, -4.859) -> (25.7735, 0.141)
  line L113 (25.7735, 0.141) -> (22.8868, 5.141)
  line L114 (27.1132, 12.4615) -> (32.8868, 12.4615)
  line L115 (24.2265, 17.4615) -> (27.1132, 12.4615)
  line L116 (27.1132, 22.4615) -> (24.2265, 17.4615)
  line L117 (32.8868, 22.4615) -> (27.1132, 22.4615)
  line L118 (32.8868, 12.4615) -> (35.7735, 17.4615)
  line L119 (35.7735, 17.4615) -> (32.8868, 22.4615)
  line L120 (37.1132, 29.782) -> (42.8868, 29.782)
  line L121 (34.2265, 34.782) -> (37.1132, 29.782)
  line L122 (37.1132, 39.782) -> (34.2265, 34.782)
  line L123 (42.8868, 29.782) -> (45.7735, 34.782)
  line L124 (45.7735, 34.782) -> (42.8868, 39.782)
  line L125 (-7.1132, -35.3205) -> (-12.8868, -35.3205)
  line L126 (-2.8868, -28) -> (2.8868, -28)
  line L127 (-5.7735, -23) -> (-2.8868, -28)
  line L128 (-2.8868, -18) -> (-5.7735, -23)
  line L129 (2.8868, -18) -> (-2.8868, -18)
  line L130 (2.8868, -28) -> (5.7735, -23)
  line L131 (5.7735, -23) -> (2.8868, -18)
  line L132 (7.1132, -10.6795) -> (12.8868, -10.6795)
  line L133 (4.2265, -5.6795) -> (7.1132, -10.6795)
  line L134 (7.1132, -0.6795) -> (4.2265, -5.6795)
  line L135 (12.8868, -0.6795) -> (7.1132, -0.6795)
  line L136 (12.8868, -10.6795) -> (15.7735, -5.6795)
  line L137 (15.7735, -5.6795) -> (12.8868, -0.6795)
  line L138 (17.1132, 6.641) -> (22.8868, 6.641)
  line L139 (14.2265, 11.641) -> (17.1132, 6.641)
  line L140 (17.1132, 16.641) -> (14.2265, 11.641)
  line L141 (22.8868, 16.641) -> (17.1132, 16.641)
  line L142 (22.8868, 6.641) -> (25.7735, 11.641)
  line L143 (25.7735, 11.641) -> (22.8868, 16.641)
  line L144 (27.1132, 23.9615) -> (32.8868, 23.9615)
  line L145 (24.2265, 28.9615) -> (27.1132, 23.9615)
  line L146 (27.1132, 33.9615) -> (24.2265, 28.9615)
  line L147 (32.8868, 33.9615) -> (27.1132, 33.9615)
  line L148 (32.8868, 23.9615) -> (35.7735, 28.9615)
  line L149 (35.7735, 28.9615) -> (32.8868, 33.9615)
  line L150 (-12.8868, -33.8205) -> (-7.1132, -33.8205)
  line L151 (-15.7735, -28.8205) -> (-12.8868, -33.8205)
  line L152 (-12.8868, -23.8205) -> (-15.7735, -28.8205)
  line L153 (-7.1132, -23.8205) -> (-12.8868, -23.8205)
  line L154 (-7.1132, -33.8205) -> (-4.2265, -28.8205)
  line L155 (-4.2265, -28.8205) -> (-7.1132, -23.8205)
  line L156 (-2.8868, -16.5) -> (2.8868, -16.5)
  line L157 (-5.7735, -11.5) -> (-2.8868, -16.5)
  line L158 (-2.8868, -6.5) -> (-5.7735, -11.5)
  line L159 (2.8868, -6.5) -> (-2.8868, -6.5)
  line L160 (2.8868, -16.5) -> (5.7735, -11.5)
  line L161 (5.7735, -11.5) -> (2.8868, -6.5)
  line L162 (7.1132, 0.8205) -> (12.8868, 0.8205)
  line L163 (4.2265, 5.8205) -> (7.1132, 0.8205)
  line L164 (7.1132, 10.8205) -> (4.2265, 5.8205)
  line L165 (12.8868, 10.8205) -> (7.1132, 10.8205)
  line L166 (12.8868, 0.8205) -> (15.7735, 5.8205)
  line L167 (15.7735, 5.8205) -> (12.8868, 10.8205)
  line L168 (17.1132, 18.141) -> (22.8868, 18.141)
  line L169 (14.2265, 23.141) -> (17.1132, 18.141)
  line L170 (17.1132, 28.141) -> (14.2265, 23.141)
  line L171 (22.8868, 28.141) -> (17.1132, 28.141)
  line L172 (22.8868, 18.141) -> (25.7735, 23.141)
  line L173 (25.7735, 23.141) -> (22.8868, 28.141)
  line L174 (27.1132, 35.4615) -> (32.8868, 35.4615)
  line L175 (24.2265, 40.4615) -> (27.1132, 35.4615)
  line L176 (32.8868, 35.4615) -> (35.7735, 40.4615)
  line L177 (-22.8868, -29.641) -> (-25.7735, -34.641)
  line L178 (-17.1132, -29.641) -> (-22.8868, -29.641)
  line L179 (-14.2265, -34.641) -> (-17.1132, -29.641)
  line L180 (-12.8868, -22.3205) -> (-7.1132, -22.3205)
  line L181 (-15.7735, -17.3205) -> (-12.8868, -22.3205)
  line L182 (-12.8868, -12.3205) -> (-15.7735, -17.3205)
  line L183 (-7.1132, -12.3205) -> (-12.8868, -12.3205)
  line L184 (-7.1132, -22.3205) -> (-4.2265, -17.3205)
  line L185 (-4.2265, -17.3205) -> (-7.1132, -12.3205)
  line L186 (7.1132, 12.3205) -> (12.8868, 12.3205)
  line L187 (4.2265, 17.3205) -> (7.1132, 12.3205)
  line L188 (7.1132, 22.3205) -> (4.2265, 17.3205)
  line L189 (12.8868, 22.3205) -> (7.1132, 22.3205)
  line L190 (12.8868, 12.3205) -> (15.7735, 17.3205)
  line L191 (15.7735, 17.3205) -> (12.8868, 22.3205)
  line L192 (17.1132, 29.641) -> (22.8868, 29.641)
  line L193 (14.2265, 34.641) -> (17.1132, 29.641)
  line L194 (17.1132, 39.641) -> (14.2265, 34.641)
  line L195 (22.8868, 29.641) -> (25.7735, 34.641)
  line L196 (25.7735, 34.641) -> (22.8868, 39.641)
  line L197 (-27.1132, -35.4615) -> (-32.8868, -35.4615)
  line L198 (-22.8868, -28.141) -> (-17.1132, -28.141)
  line L199 (-25.7735, -23.141) -> (-22.8868, -28.141)
  line L200 (-22.8868, -18.141) -> (-25.7735, -23.141)
  line L201 (-17.1132, -18.141) -> (-22.8868, -18.141)
  line L202 (-17.1132, -28.141) -> (-14.2265, -23.141)
  line L203 (-14.2265, -23.141) -> (-17.1132, -18.141)
  line L204 (-12.8868, -10.8205) -> (-7.1132, -10.8205)
  line L205 (-15.7735, -5.8205) -> (-12.8868, -10.8205)
  line L206 (-12.8868, -0.8205) -> (-15.7735, -5.8205)
  line L207 (-7.1132, -0.8205) -> (-12.8868, -0.8205)
  line L208 (-7.1132, -10.8205) -> (-4.2265, -5.8205)
  line L209 (-4.2265, -5.8205) -> (-7.1132, -0.8205)
  line L210 (-2.8868, 6.5) -> (2.8868, 6.5)
  line L211 (-5.7735, 11.5) -> (-2.8868, 6.5)
  line L212 (-2.8868, 16.5) -> (-5.7735, 11.5)
  line L213 (2.8868, 16.5) -> (-2.8868, 16.5)
  line L214 (2.8868, 6.5) -> (5.7735, 11.5)
  line L215 (5.7735, 11.5) -> (2.8868, 16.5)
  line L216 (7.1132, 23.8205) -> (12.8868, 23.8205)
  line L217 (4.2265, 28.8205) -> (7.1132, 23.8205)
  line L218 (7.1132, 33.8205) -> (4.2265, 28.8205)
  line L219 (12.8868, 33.8205) -> (7.1132, 33.8205)
  line L220 (12.8868, 23.8205) -> (15.7735, 28.8205)
  line L221 (15.7735, 28.8205) -> (12.8868, 33.8205)
  line L222 (-32.8868, -33.9615) -> (-27.1132, -33.9615)
  line L223 (-35.7735, -28.9615) -> (-32.8868, -33.9615)
  line L224 (-32.8868, -23.9615) -> (-35.7735, -28.9615)
  line L225 (-27.1132, -23.9615) -> (-32.8868, -23.9615)
  line L226 (-27.1132, -33.9615) -> (-24.2265, -28.9615)
  line L227 (-24.2265, -28.9615) -> (-27.1132, -23.9615)
  line L228 (-22.8868, -16.641) -> (-17.1132, -16.641)
  line L229 (-25.7735, -11.641) -> (-22.8868, -16.641)
  line L230 (-22.8868, -6.641) -> (-25.7735, -11.641)
  line L231 (-17.1132, -6.641) -> (-22.8868, -6.641)
  line L232 (-17.1132, -16.641) -> (-14.2265, -11.641)
  line L233 (-14.2265, -11.641) -> (-17.1132, -6.641)
  line L234 (-12.8868, 0.6795) -> (-7.1132, 0.6795)
  line L235 (-15.7735, 5.6795) -> (-12.8868, 0.6795)
  line L236 (-12.8868, 10.6795) -> (-15.7735, 5.6795)
  line L237 (-7.1132, 10.6795) -> (-12.8868, 10.6795)
  line L238 (-7.1132, 0.6795) -> (-4.2265, 5.6795)
  line L239 (-4.2265, 5.6795) -> (-7.1132, 10.6795)
  line L240 (-2.8868, 18) -> (2.8868, 18)
  line L241 (-5.7735, 23) -> (-2.8868, 18)
  line L242 (-2.8868, 28) -> (-5.7735, 23)
  line L243 (2.8868, 28) -> (-2.8868, 28)
  line L244 (2.8868, 18) -> (5.7735, 23)
  line L245 (5.7735, 23) -> (2.8868, 28)
  line L246 (7.1132, 35.3205) -> (12.8868, 35.3205)
  line L247 (4.2265, 40.3205) -> (7.1132, 35.3205)
  line L248 (12.8868, 35.3205) -> (15.7735, 40.3205)
  line L249 (-42.8868, -29.782) -> (-45.7735, -34.782)
  line L250 (-37.1132, -29.782) -> (-42.8868, -29.782)
  line L251 (-34.2265, -34.782) -> (-37.1132, -29.782)
  line L252 (-32.8868, -22.4615) -> (-27.1132, -22.4615)
  line L253 (-35.7735, -17.4615) -> (-32.8868, -22.4615)
  line L254 (-32.8868, -12.4615) -> (-35.7735, -17.4615)
  line L255 (-27.1132, -12.4615) -> (-32.8868, -12.4615)
  line L256 (-27.1132, -22.4615) -> (-24.2265, -17.4615)
  line L257 (-24.2265, -17.4615) -> (-27.1132, -12.4615)
  line L258 (-22.8868, -5.141) -> (-17.1132, -5.141)
  line L259 (-25.7735, -0.141) -> (-22.8868, -5.141)
  line L260 (-22.8868, 4.859) -> (-25.7735, -0.141)
  line L261 (-17.1132, 4.859) -> (-22.8868, 4.859)
  line L262 (-17.1132, -5.141) -> (-14.2265, -0.141)
  line L263 (-14.2265, -0.141) -> (-17.1132, 4.859)
  line L264 (-12.8868, 12.1795) -> (-7.1132, 12.1795)
  line L265 (-15.7735, 17.1795) -> (-12.8868, 12.1795)
  line L266 (-12.8868, 22.1795) -> (-15.7735, 17.1795)
  line L267 (-7.1132, 22.1795) -> (-12.8868, 22.1795)
  line L268 (-7.1132, 12.1795) -> (-4.2265, 17.1795)
  line L269 (-4.2265, 17.1795) -> (-7.1132, 22.1795)
  line L270 (-2.8868, 29.5) -> (2.8868, 29.5)
  line L271 (-5.7735, 34.5) -> (-2.8868, 29.5)
  line L272 (-2.8868, 39.5) -> (-5.7735, 34.5)
  line L273 (2.8868, 29.5) -> (5.7735, 34.5)
  line L274 (5.7735, 34.5) -> (2.8868, 39.5)
  line L275 (-42.8868, -28.282) -> (-37.1132, -28.282)
  line L276 (-45.7735, -23.282) -> (-42.8868, -28.282)
  line L277 (-42.8868, -18.282) -> (-45.7735, -23.282)
  line L278 (-37.1132, -18.282) -> (-42.8868, -18.282)
  line L279 (-37.1132, -28.282) -> (-34.2265, -23.282)
  line L280 (-34.2265, -23.282) -> (-37.1132, -18.282)
  line L281 (-32.8868, -10.9615) -> (-27.1132, -10.9615)
  line L282 (-35.7735, -5.9615) -> (-32.8868, -10.9615)
  line L283 (-32.8868, -0.9615) -> (-35.7735, -5.9615)
  line L284 (-27.1132, -0.9615) -> (-32.8868, -0.9615)
  line L285 (-27.1132, -10.9615) -> (-24.2265, -5.9615)
  line L286 (-24.2265, -5.9615) -> (-27.1132, -0.9615)
  line L287 (-22.8868, 6.359) -> (-17.1132, 6.359)
  line L288 (-25.7735, 11.359) -> (-22.8868, 6.359)
  line L289 (-22.8868, 16.359) -> (-25.7735, 11.359)
  line L290 (-17.1132, 16.359) -> (-22.8868, 16.359)
  line L291 (-17.1132, 6.359) -> (-14.2265, 11.359)
  line L292 (-14.2265, 11.359) -> (-17.1132, 16.359)
  line L293 (-12.8868, 23.6795) -> (-7.1132, 23.6795)
  line L294 (-15.7735, 28.6795) -> (-12.8868, 23.6795)
  line L295 (-12.8868, 33.6795) -> (-15.7735, 28.6795)
  line L296 (-7.1132, 33.6795) -> (-12.8868, 33.6795)
  line L297 (-7.1132, 23.6795) -> (-4.2265, 28.6795)
  line L298 (-4.2265, 28.6795) -> (-7.1132, 33.6795)
  line L299 (-42.8868, -16.782) -> (-37.1132, -16.782)
  line L300 (-45.7735, -11.782) -> (-42.8868, -16.782)
  line L301 (-42.8868, -6.782) -> (-45.7735, -11.782)
  line L302 (-37.1132, -6.782) -> (-42.8868, -6.782)
  line L303 (-37.1132, -16.782) -> (-34.2265, -11.782)
  line L304 (-34.2265, -11.782) -> (-37.1132, -6.782)
  line L305 (-32.8868, 0.5385) -> (-27.1132, 0.5385)
  line L306 (-35.7735, 5.5385) -> (-32.8868, 0.5385)
  line L307 (-32.8868, 10.5385) -> (-35.7735, 5.5385)
  line L308 (-27.1132, 10.5385) -> (-32.8868, 10.5385)
  line L309 (-27.1132, 0.5385) -> (-24.2265, 5.5385)
  line L310 (-24.2265, 5.5385) -> (-27.1132, 10.5385)
  line L311 (-22.8868, 17.859) -> (-17.1132, 17.859)
  line L312 (-25.7735, 22.859) -> (-22.8868, 17.859)
  line L313 (-22.8868, 27.859) -> (-25.7735, 22.859)
  line L314 (-17.1132, 27.859) -> (-22.8868, 27.859)
  line L315 (-17.1132, 17.859) -> (-14.2265, 22.859)
  line L316 (-14.2265, 22.859) -> (-17.1132, 27.859)
  line L317 (-12.8868, 35.1795) -> (-7.1132, 35.1795)
  line L318 (-15.7735, 40.1795) -> (-12.8868, 35.1795)
  line L319 (-7.1132, 35.1795) -> (-4.2265, 40.1795)
  line L320 (-42.8868, -5.282) -> (-37.1132, -5.282)
  line L321 (-45.7735, -0.282) -> (-42.8868, -5.282)
  line L322 (-42.8868, 4.718) -> (-45.7735, -0.282)
  line L323 (-37.1132, 4.718) -> (-42.8868, 4.718)
  line L324 (-37.1132, -5.282) -> (-34.2265, -0.282)
  line L325 (-34.2265, -0.282) -> (-37.1132, 4.718)
  line L326 (-32.8868, 12.0385) -> (-27.1132, 12.0385)
  line L327 (-35.7735, 17.0385) -> (-32.8868, 12.0385)
  line L328 (-32.8868, 22.0385) -> (-35.7735, 17.0385)
  line L329 (-27.1132, 22.0385) -> (-32.8868, 22.0385)
  line L330 (-27.1132, 12.0385) -> (-24.2265, 17.0385)
  line L331 (-24.2265, 17.0385) -> (-27.1132, 22.0385)
  line L332 (-22.8868, 29.359) -> (-17.1132, 29.359)
  line L333 (-25.7735, 34.359) -> (-22.8868, 29.359)
  line L334 (-22.8868, 39.359) -> (-25.7735, 34.359)
  line L335 (-17.1132, 29.359) -> (-14.2265, 34.359)
  line L336 (-14.2265, 34.359) -> (-17.1132, 39.359)
  line L337 (-42.8868, 6.218) -> (-37.1132, 6.218)
  line L338 (-45.7735, 11.218) -> (-42.8868, 6.218)
  line L339 (-42.8868, 16.218) -> (-45.7735, 11.218)
  line L340 (-37.1132, 16.218) -> (-42.8868, 16.218)
  line L341 (-37.1132, 6.218) -> (-34.2265, 11.218)
  line L342 (-34.2265, 11.218) -> (-37.1132, 16.218)
  line L343 (-32.8868, 23.5385) -> (-27.1132, 23.5385)
  line L344 (-35.7735, 28.5385) -> (-32.8868, 23.5385)
  line L345 (-32.8868, 33.5385) -> (-35.7735, 28.5385)
  line L346 (-27.1132, 33.5385) -> (-32.8868, 33.5385)
  line L347 (-27.1132, 23.5385) -> (-24.2265, 28.5385)
  line L348 (-24.2265, 28.5385) -> (-27.1132, 33.5385)
  line L349 (-42.8868, 17.718) -> (-37.1132, 17.718)
  line L350 (-45.7735, 22.718) -> (-42.8868, 17.718)
  line L351 (-42.8868, 27.718) -> (-45.7735, 22.718)
  line L352 (-37.1132, 27.718) -> (-42.8868, 27.718)
  line L353 (-37.1132, 17.718) -> (-34.2265, 22.718)
  line L354 (-34.2265, 22.718) -> (-37.1132, 27.718)
  line L355 (-32.8868, 35.0385) -> (-27.1132, 35.0385)
  line L356 (-35.7735, 40.0385) -> (-32.8868, 35.0385)
  line L357 (-27.1132, 35.0385) -> (-24.2265, 40.0385)
  arc A11 (-40.0874, -27.5026) -> (-34.5883, -32.9025) centre (-34.5883, -27.4025) ccw
  line L358 (-40.0874, -27.5026) -> (-40.1132, -26.0867)
  arc A12 (-40.1132, -26.0867) -> (-44.6124, -21.6685) centre (-44.6124, -26.1685) ccw
  line L359 (-44.6124, -21.6685) -> (-65.104, -21.6685)
  arc A13 (-70.604, -16.1685) -> (-65.104, -21.6685) centre (-65.104, -16.1685) ccw
  line L360 (-70.604, -16.1685) -> (-70.604, 27.4032)
  arc A14 (-65.104, 32.9032) -> (-70.604, 27.4032) centre (-65.104, 27.4032) ccw
  line L361 (-65.104, 32.9032) -> (65.104, 32.9032)
  arc A15 (70.604, 27.4032) -> (65.104, 32.9032) centre (65.104, 27.4032) ccw
  line L362 (70.604, 27.4032) -> (70.604, -16.1685)
  arc A16 (65.104, -21.6685) -> (70.604, -16.1685) centre (65.104, -16.1685) ccw
  line L363 (65.104, -21.6685) -> (44.6124, -21.6685)
  arc A17 (44.6124, -21.6685) -> (40.1132, -26.0867) centre (44.6124, -26.1685) ccw
  line L364 (40.1132, -26.0867) -> (40.0874, -27.5026)
  arc A18 (34.5883, -32.9025) -> (40.0874, -27.5026) centre (34.5883, -27.4025) ccw
  line L365 (34.5883, -32.9025) -> (-34.5883, -32.9025)
  arc A19 (34.5883, -35.9025) -> (43.0869, -27.5571) centre (34.5883, -27.4025) ccw
  line L366 (43.0869, -27.5571) -> (43.1127, -26.1412)
  arc A20 (44.6124, -24.6685) -> (43.1127, -26.1412) centre (44.6124, -26.1685) ccw
  line L367 (44.6124, -24.6685) -> (65.104, -24.6685)
  arc A21 (65.104, -24.6685) -> (73.604, -16.1685) centre (65.104, -16.1685) ccw
  line L368 (73.604, -16.1685) -> (73.604, 27.4032)
  arc A22 (73.604, 27.4032) -> (65.104, 35.9032) centre (65.104, 27.4032) ccw
  line L369 (65.104, 35.9032) -> (-65.104, 35.9032)
  arc A23 (-65.104, 35.9032) -> (-73.604, 27.4032) centre (-65.104, 27.4032) ccw
  line L370 (-73.604, 27.4032) -> (-73.604, -16.1685)
  arc A24 (-73.604, -16.1685) -> (-65.104, -24.6685) centre (-65.104, -16.1685) ccw
  line L371 (-65.104, -24.6685) -> (-44.6124, -24.6685)
  arc A25 (-43.1127, -26.1412) -> (-44.6124, -24.6685) centre (-44.6124, -26.1685) ccw
  line L372 (-43.1127, -26.1412) -> (-43.0869, -27.5571)
  arc A26 (-43.0869, -27.5571) -> (-34.5883, -35.9025) centre (-34.5883, -27.4025) ccw
  line L373 (-34.5883, -35.9025) -> (34.5883, -35.9025)
  arc A27 (-35.0882, -27.4116) -> (-34.5883, -27.9025) centre (-34.5883, -27.4025) ccw
  line L374 (34.5883, -27.9025) -> (-34.5883, -27.9025)
  arc A28 (34.5883, -27.9025) -> (35.0882, -27.4116) centre (34.5883, -27.4025) ccw
  line L375 (35.114, -25.9957) -> (35.0882, -27.4116)
  arc A29 (44.6124, -16.6685) -> (35.114, -25.9957) centre (44.6124, -26.1685) ccw
  line L376 (65.104, -16.6685) -> (44.6124, -16.6685)
  arc A30 (65.104, -16.6685) -> (65.604, -16.1685) centre (65.104, -16.1685) ccw
  line L377 (65.604, 27.4032) -> (65.604, -16.1685)
  arc A31 (65.604, 27.4032) -> (65.104, 27.9032) centre (65.104, 27.4032) ccw
  line L378 (-65.104, 27.9032) -> (65.104, 27.9032)
  arc A32 (-65.104, 27.9032) -> (-65.604, 27.4032) centre (-65.104, 27.4032) ccw
  line L379 (-65.604, -16.1685) -> (-65.604, 27.4032)
  arc A33 (-65.604, -16.1685) -> (-65.104, -16.6685) centre (-65.104, -16.1685) ccw
  line L380 (-44.6124, -16.6685) -> (-65.104, -16.6685)
  arc A34 (-35.114, -25.9957) -> (-44.6124, -16.6685) centre (-44.6124, -26.1685) ccw
  line L381 (-35.0882, -27.4116) -> (-35.114, -25.9957)
  line L382 (-30, 33.5385) -> (-30, -5.1548)
  arc A35 (-32.5288, -8.1176) -> (-41.8158, -17.0895) centre (-30.7597, -19.2414) ccw
  arc A36 (-32.5288, -8.1176) -> (-30, -5.1548) centre (-33, -5.1548) ccw
  line L383 (-0.0002, -46.8087) -> (-0.0002, -40)
  arc A37 (41.8154, -17.0895) -> (32.5284, -8.1176) centre (30.7593, -19.2414) ccw
  line L384 (29.9996, 33.5385) -> (29.9996, -5.1548)
  arc A38 (29.9996, -5.1548) -> (32.5284, -8.1176) centre (32.9996, -5.1548) ccw
  line L385 (25.9996, 33.5385) -> (25.9996, -5.1548)
  arc A39 (25.9996, -5.1548) -> (31.9002, -12.068) centre (32.9996, -5.1548) ccw
  arc A40 (37.8891, -17.8537) -> (31.9002, -12.068) centre (30.7593, -19.2414) ccw
  line L386 (-37.8895, -17.8537) -> (-37.9563, -19.3902)
  line L387 (37.8891, -17.8537) -> (37.9563, -19.3902)
  line L388 (30, -32.9025) -> (30, 32.9032)
  arc A41 (-32, -9) -> (-42, -19) centre (-32, -19) ccw
  line L389 (-32, -9) -> (-31, -9)